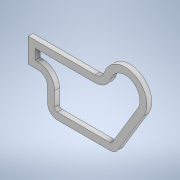
# Autodesk Inventor part: ch6-gasket
Saved by Autodesk Inventor 2020 (Build 240168000, 168)
## iProperties
Created: 2020-02-21
Part Number: ch6-gasket
Material: Generic
Document SubType Name: Modeling
Designer: Eric
Density: 1 g/cm^3
Appearance: Default
Author: Eric
Autodesk Inventor part; units mm, degrees
ref_plane "YZ Plane" through (0, 0, 0) normal (1, 0, 0) x (0, 1, 0)
ref_plane "XZ Plane" through (0, 0, 0) normal (0, 1, 0) x (-1, 0, 0)
ref_plane "XY Plane" through (0, 0, 0) normal (0, 0, 1) x (1, 0, 0)
sketch "Sketch1" plane through (0, 0, 0) normal (0, 0, 1) x (1, 0, 0)
  line L0 (-58.4714, 122.8857) -> (-58.4714, 72.8857)
  line L1 (-58.4714, 72.8857) -> (-38.4714, 72.8857)
  line L2 (-18.4714, 52.8857) -> (-18.4714, 22.8857)
  line L3 (1.5286, 2.8857) -> (110.2526, 2.8857)
  line L4 (127.365, 12.5337) -> (180.0315, 99.5936)
  line L5 (-58.4714, 122.8857) -> (96.5286, 122.8857)
  circle A0 centre (141.5286, 122.8857) radius 45
  arc A1 (-18.4714, 52.8857) -> (-38.4714, 72.8857) centre (-38.4714, 52.8857) ccw
  arc A2 (-18.4714, 22.8857) -> (1.5286, 2.8857) centre (1.5286, 22.8857) ccw
  arc A3 (110.2526, 2.8857) -> (127.365, 12.5337) centre (110.2526, 22.8857) ccw
  circle A4 centre (79.682, 142.8857) radius 20
  line L6 (332.4097, 149.7121) -> (512.4097, 149.7121)
  line L7 (512.4097, 149.7121) -> (512.4097, 29.7121)
  line L8 (512.4097, 29.7121) -> (332.4097, 29.7121)
  line L9 (332.4097, 29.7121) -> (332.4097, 149.7121)
  circle A5 centre (512.4097, 149.7121) radius 54.8405
  point P0 (0, 0)
  point P1 (-18.4714, 72.8857)
  point P2 (-18.4714, 2.8857)
  point P3 (121.5286, 2.8857)
  point P4 (512.4097, 94.8716)
  point P5 (457.5692, 149.7121)
  point P6 (98.7117, 136.7319)
  point P7 (79.682, 122.8857)
  dimension "WIDTH" = 120
  dimension "LENGTH" = 180
  dimension "d2" = 200
  dimension "d3" = 40
  dimension "d4" = 50
  dimension "d5" = 20
  dimension "d6" = 40
  dimension "d7" = 90
  dimension "d8" = 180
  dimension "d9" = 120
  constraints: 20 end point, 9 tangent, 8 point on circle, 6 centre point, 6 point on line, 3 horizontal, 3 perpendicular, 2 equal radius, 2 parallel, 1 coincident, 1 horizontal alignment, 1 vertical
  measures "WIDTH" vertical distance of point (-18.471, 2.886) L0.start
  measures "LENGTH" horizontal distance of point (121.529, 2.886) L0.end
  measures "d2" distance of A0.centre L0.start
  measures "d3" distance of L0.end point (-18.471, 72.886)
  measures "d4" distance of L0.start L0.end
  measures "d5" radius of A1
  measures "d6" diameter of A4
  measures "d7" diameter of A0
  measures "d8" distance of L7.end L8.end
  measures "d9" distance of L8.end L6.start
extrude "Extrusion1" add sketch "Sketch1" along normal blind 10 contours L5 A0 L4 A3 L3 A2 L2 A1 L1 L0 | A4 A0 L5 | A0
sketch "Sketch3" plane through (0, 0, 10) normal (0, 0, 1) x (1, 0, 0)
  line L0 (-18.4714, 52.8857) -> (-18.4714, 22.8857) projected
  arc A0 (-18.4714, 22.8857) -> (1.5286, 2.8857) centre (1.5286, 22.8857) ccw projected
  line L1 (1.5286, 2.8857) -> (110.2526, 2.8857) projected
  arc A1 (110.2526, 2.8857) -> (127.365, 12.5337) centre (110.2526, 22.8857) ccw projected
  line L2 (127.365, 12.5337) -> (180.0315, 99.5936) projected
  arc A2 (180.0315, 99.5936) -> (98.7117, 136.7319) centre (141.5286, 122.8857) ccw projected
  arc A3 (79.682, 122.8857) -> (98.7117, 136.7319) centre (79.682, 142.8857) ccw projected
  line L3 (79.682, 122.8857) -> (-58.4714, 122.8857) projected
  line L4 (-58.4714, 122.8857) -> (-58.4714, 72.8857) projected
  line L5 (-58.4714, 72.8857) -> (-38.4714, 72.8857) projected
  arc A4 (-18.4714, 52.8857) -> (-38.4714, 72.8857) centre (-38.4714, 52.8857) ccw projected
  line L6 (-44.1571, 108.5714) -> (79.682, 108.5714)
  arc A5 (79.682, 108.5714) -> (112.3315, 132.3275) centre (79.682, 142.8857) ccw
  arc A6 (167.7839, 107.0027) -> (112.3315, 132.3275) centre (141.5286, 122.8857) ccw
  line L7 (167.7839, 107.0027) -> (115.1175, 19.9428)
  arc A7 (110.2526, 17.2) -> (115.1175, 19.9428) centre (110.2526, 22.8857) ccw
  line L8 (110.2526, 17.2) -> (1.5286, 17.2)
  arc A8 (-4.1571, 22.8857) -> (1.5286, 17.2) centre (1.5286, 22.8857) ccw
  line L9 (-4.1571, 22.8857) -> (-4.1571, 52.8857)
  arc A9 (-4.1571, 52.8857) -> (-38.4714, 87.2) centre (-38.4714, 52.8857) ccw
  line L10 (-38.4714, 87.2) -> (-44.1571, 87.2)
  line L11 (-44.1571, 87.2) -> (-44.1571, 108.5714)
  point P0 (0, 0)
  constraints: 12 end point, 10 point on circle, 5 centre point, 10 other
extrude "Extrusion3" cut sketch "Sketch3" against normal through all contours L6 A5 A6 L7 A7 L8 A8 L9 A9 L10 L11
equation "\"d8\" = LENGTH"
equation "\"d9\" = WIDTH"
body "Solid1"
